Autodesk Fusion 360 part; units mm, degrees
(part 11 of 15)
  spline S48 degree 5 poles (7.9532, 21.0514) (7.9591, 21.034) (7.9709, 20.999) (7.9884, 20.9466) (8.0117, 20.8767) (8.0404, 20.7893) (8.0688, 20.7018) (8.0969, 20.6143) (8.1247, 20.5268) (8.1522, 20.4393) (8.1794, 20.3517) (8.2063, 20.2641) (8.2329, 20.1765) (8.2592, 20.0889) (8.2851, 20.0012) (8.3107, 19.9135) (8.336, 19.8258) (8.361, 19.7381) (8.3856, 19.6503) (8.41, 19.5626) (8.4339, 19.4747) (8.4576, 19.3869) (8.4809, 19.2991) (8.5039, 19.2112) (8.5265, 19.1233) (8.5488, 19.0354) (8.5707, 18.9475) (8.5923, 18.8596) (8.6135, 18.7716) (8.6343, 18.6836) (8.6548, 18.5957) (8.675, 18.5077) (8.6947, 18.4196) (8.7141, 18.3316) (8.7331, 18.2436) (8.7517, 18.1555) (8.7699, 18.0674) (8.7878, 17.9794) (8.8052, 17.8913) (8.8222, 17.8032) (8.8388, 17.7151) (8.855, 17.627) (8.8695, 17.5461) (8.8806, 17.4828) (8.8884, 17.4371) (8.8932, 17.409) (8.895, 17.3986) knots -1 -1 -1 -1 -1 -1 -0.985714 -0.971429 -0.957143 -0.942857 -0.928571 -0.914286 -0.9 -0.885714 -0.871429 -0.857143 -0.842857 -0.828571 -0.814286 -0.8 -0.785714 -0.771429 -0.757143 -0.742857 -0.728571 -0.714286 -0.7 -0.685714 -0.671429 -0.657143 -0.642857 -0.628571 -0.614286 -0.6 -0.585714 -0.571429 -0.557143 -0.542857 -0.528571 -0.514286 -0.5 -0.485714 -0.471429 -0.457143 -0.442857 -0.428571 -0.414286 -0.405839 -0.405839 -0.405839 -0.405839 -0.405839 -0.405839
  arc A48 (10.2055, 17.2577) -> (8.895, 17.3986) centre (2.0032, -52.8695) ccw
  spline S49 degree 5 poles (10.2055, 17.2577) (10.2095, 17.2675) (10.2201, 17.2939) (10.2374, 17.3369) (10.2617, 17.3964) (10.2931, 17.4724) (10.3276, 17.555) (10.3626, 17.6376) (10.398, 17.72) (10.4337, 17.8024) (10.4699, 17.8847) (10.5064, 17.9669) (10.5433, 18.0489) (10.5806, 18.1309) (10.6182, 18.2128) (10.6562, 18.2946) (10.6946, 18.3764) (10.7333, 18.458) (10.7724, 18.5395) (10.8118, 18.6209) (10.8516, 18.7023) (10.8917, 18.7835) (10.9322, 18.8647) (10.973, 18.9458) (11.0141, 19.0267) (11.0555, 19.1076) (11.0973, 19.1884) (11.1394, 19.2691) (11.1818, 19.3497) (11.2246, 19.4302) (11.2676, 19.5106) (11.311, 19.591) (11.3547, 19.6712) (11.3986, 19.7514) (11.4429, 19.8314) (11.4875, 19.9114) (11.5324, 19.9913) (11.5776, 20.071) (11.6231, 20.1507) (11.6689, 20.2303) (11.7149, 20.3098) (11.7613, 20.3892) (11.808, 20.4685) (11.8455, 20.5319) (11.8738, 20.5794) (11.8927, 20.6111) (11.9022, 20.6269) knots 0.405839 0.405839 0.405839 0.405839 0.405839 0.405839 0.414286 0.428571 0.442857 0.457143 0.471429 0.485714 0.5 0.514286 0.528571 0.542857 0.557143 0.571429 0.585714 0.6 0.614286 0.628571 0.642857 0.657143 0.671429 0.685714 0.7 0.714286 0.728571 0.742857 0.757143 0.771429 0.785714 0.8 0.814286 0.828571 0.842857 0.857143 0.871429 0.885714 0.9 0.914286 0.928571 0.942857 0.957143 0.971429 0.985714 1 1 1 1 1 1
  arc A49 (13.2115, 20.4386) -> (11.9022, 20.6269) centre (2.0032, -52.8695) ccw
  spline S50 degree 5 poles (13.2115, 20.4386) (13.2162, 20.4208) (13.2254, 20.3851) (13.2392, 20.3316) (13.2573, 20.2602) (13.2798, 20.1709) (13.3019, 20.0817) (13.3237, 19.9924) (13.3452, 19.9031) (13.3664, 19.8138) (13.3873, 19.7246) (13.4078, 19.6353) (13.4281, 19.546) (13.448, 19.4567) (13.4676, 19.3674) (13.4869, 19.2781) (13.5059, 19.1888) (13.5246, 19.0995) (13.5429, 19.0102) (13.5609, 18.921) (13.5785, 18.8317) (13.5959, 18.7424) (13.6128, 18.6531) (13.6295, 18.5638) (13.6458, 18.4745) (13.6617, 18.3853) (13.6773, 18.296) (13.6926, 18.2068) (13.7075, 18.1175) (13.722, 18.0283) (13.7361, 17.9391) (13.7499, 17.8498) (13.7634, 17.7606) (13.7764, 17.6714) (13.7891, 17.5823) (13.8014, 17.4931) (13.8133, 17.404) (13.8248, 17.3149) (13.8359, 17.2257) (13.8466, 17.1367) (13.8569, 17.0476) (13.8667, 16.9586) (13.8754, 16.8768) (13.882, 16.8129) (13.8865, 16.7668) (13.8893, 16.7385) (13.8903, 16.7279) knots -1 -1 -1 -1 -1 -1 -0.985714 -0.971429 -0.957143 -0.942857 -0.928571 -0.914286 -0.9 -0.885714 -0.871429 -0.857143 -0.842857 -0.828571 -0.814286 -0.8 -0.785714 -0.771429 -0.757143 -0.742857 -0.728571 -0.714286 -0.7 -0.685714 -0.671429 -0.657143 -0.642857 -0.628571 -0.614286 -0.6 -0.585714 -0.571429 -0.557143 -0.542857 -0.528571 -0.514286 -0.5 -0.485714 -0.471429 -0.457143 -0.442857 -0.428571 -0.414286 -0.405839 -0.405839 -0.405839 -0.405839 -0.405839 -0.405839
  arc A50 (15.1874, 16.4939) -> (13.8903, 16.7279) centre (2.0032, -52.8695) ccw
  spline S51 degree 5 poles (15.1874, 16.4939) (15.1921, 16.5034) (15.2045, 16.529) (15.2249, 16.5706) (15.2534, 16.6282) (15.2901, 16.7018) (15.3305, 16.7817) (15.3712, 16.8616) (15.4124, 16.9413) (15.4539, 17.0209) (15.4958, 17.1004) (15.5381, 17.1798) (15.5808, 17.259) (15.6238, 17.3381) (15.6672, 17.4171) (15.711, 17.496) (15.7551, 17.5748) (15.7995, 17.6534) (15.8443, 17.732) (15.8895, 17.8104) (15.9349, 17.8887) (15.9808, 17.9669) (16.0269, 18.0449) (16.0734, 18.1229) (16.1202, 18.2007) (16.1673, 18.2784) (16.2147, 18.356) (16.2624, 18.4335) (16.3105, 18.5109) (16.3589, 18.5882) (16.4076, 18.6653) (16.4565, 18.7423) (16.5058, 18.8193) (16.5554, 18.8961) (16.6053, 18.9728) (16.6555, 19.0493) (16.706, 19.1258) (16.7567, 19.2022) (16.8078, 19.2784) (16.8591, 19.3545) (16.9108, 19.4305) (16.9627, 19.5064) (17.0149, 19.5822) (17.0568, 19.6428) (17.0884, 19.6881) (17.1096, 19.7183) (17.1202, 19.7334) knots 0.405839 0.405839 0.405839 0.405839 0.405839 0.405839 0.414286 0.428571 0.442857 0.457143 0.471429 0.485714 0.5 0.514286 0.528571 0.542857 0.557143 0.571429 0.585714 0.6 0.614286 0.628571 0.642857 0.657143 0.671429 0.685714 0.7 0.714286 0.728571 0.742857 0.757143 0.771429 0.785714 0.8 0.814286 0.828571 0.842857 0.857143 0.871429 0.885714 0.9 0.914286 0.928571 0.942857 0.957143 0.971429 0.985714 1 1 1 1 1 1
  arc A51 (18.4127, 19.4523) -> (17.1202, 19.7334) centre (2.0032, -52.8695) ccw
  spline S52 degree 5 poles (18.4127, 19.4523) (18.4161, 19.4341) (18.4227, 19.3979) (18.4326, 19.3435) (18.4457, 19.271) (18.4617, 19.1804) (18.4774, 19.0897) (18.4927, 18.9992) (18.5078, 18.9086) (18.5226, 18.818) (18.537, 18.7275) (18.5512, 18.637) (18.565, 18.5465) (18.5786, 18.456) (18.5918, 18.3655) (18.6046, 18.2751) (18.6172, 18.1846) (18.6294, 18.0942) (18.6413, 18.0039) (18.6529, 17.9135) (18.6641, 17.8232) (18.6751, 17.7329) (18.6856, 17.6426) (18.6959, 17.5524) (18.7057, 17.4622) (18.7153, 17.372) (18.7245, 17.2819) (18.7333, 17.1918) (18.7418, 17.1017) (18.7499, 17.0116) (18.7577, 16.9216) (18.7651, 16.8317) (18.7721, 16.7417) (18.7788, 16.6518) (18.785, 16.562) (18.7909, 16.4722) (18.7964, 16.3824) (18.8015, 16.2927) (18.8063, 16.203) (18.8106, 16.1134) (18.8145, 16.0238) (18.818, 15.9343) (18.8208, 15.8522) (18.8228, 15.7879) (18.824, 15.7416) (18.8248, 15.7132) (18.825, 15.7026) knots -1 -1 -1 -1 -1 -1 -0.985714 -0.971429 -0.957143 -0.942857 -0.928571 -0.914286 -0.9 -0.885714 -0.871429 -0.857143 -0.842857 -0.828571 -0.814286 -0.8 -0.785714 -0.771429 -0.757143 -0.742857 -0.728571 -0.714286 -0.7 -0.685714 -0.671429 -0.657143 -0.642857 -0.628571 -0.614286 -0.6 -0.585714 -0.571429 -0.557143 -0.542857 -0.528571 -0.514286 -0.5 -0.485714 -0.471429 -0.457143 -0.442857 -0.428571 -0.414286 -0.405839 -0.405839 -0.405839 -0.405839 -0.405839 -0.405839
  arc A52 (20.1022, 15.3766) -> (18.825, 15.7026) centre (2.0032, -52.8695) ccw
  spline S53 degree 5 poles (20.1022, 15.3766) (20.1075, 15.3858) (20.1217, 15.4104) (20.145, 15.4504) (20.1775, 15.5059) (20.2194, 15.5766) (20.2654, 15.6535) (20.3117, 15.7303) (20.3585, 15.8068) (20.4056, 15.8833) (20.4531, 15.9596) (20.5009, 16.0357) (20.5491, 16.1117) (20.5977, 16.1876) (20.6466, 16.2633) (20.6959, 16.3388) (20.7455, 16.4143) (20.7954, 16.4895) (20.8457, 16.5647) (20.8963, 16.6397) (20.9473, 16.7145) (20.9985, 16.7892) (21.0501, 16.8638) (21.102, 16.9383) (21.1543, 17.0126) (21.2068, 17.0867) (21.2597, 17.1607) (21.3128, 17.2346) (21.3663, 17.3084) (21.42, 17.382) (21.4741, 17.4555) (21.5284, 17.5288) (21.5831, 17.602) (21.638, 17.6751) (21.6933, 17.748) (21.7488, 17.8208) (21.8046, 17.8935) (21.8607, 17.966) (21.917, 18.0384) (21.9737, 18.1107) (22.0306, 18.1828) (22.0878, 18.2548) (22.1453, 18.3267) (22.1914, 18.3841) (22.2262, 18.4271) (22.2494, 18.4557) (22.2611, 18.47) knots 0.405839 0.405839 0.405839 0.405839 0.405839 0.405839 0.414286 0.428571 0.442857 0.457143 0.471429 0.485714 0.5 0.514286 0.528571 0.542857 0.557143 0.571429 0.585714 0.6 0.614286 0.628571 0.642857 0.657143 0.671429 0.685714 0.7 0.714286 0.728571 0.742857 0.757143 0.771429 0.785714 0.8 0.814286 0.828571 0.842857 0.857143 0.871429 0.885714 0.9 0.914286 0.928571 0.942857 0.957143 0.971429 0.985714 1 1 1 1 1 1
  arc A53 (23.5303, 18.0974) -> (22.2611, 18.47) centre (2.0032, -52.8695) ccw
  spline S54 degree 5 poles (23.5303, 18.0974) (23.5323, 18.079) (23.5364, 18.0424) (23.5424, 17.9874) (23.5502, 17.9142) (23.5597, 17.8226) (23.5689, 17.7312) (23.5778, 17.6397) (23.5864, 17.5483) (23.5946, 17.4569) (23.6026, 17.3655) (23.6102, 17.2742) (23.6176, 17.183) (23.6246, 17.0918) (23.6313, 17.0006) (23.6377, 16.9095) (23.6438, 16.8184) (23.6496, 16.7273) (23.655, 16.6363) (23.6601, 16.5454) (23.6649, 16.4545) (23.6693, 16.3637) (23.6734, 16.2729) (23.6772, 16.1821) (23.6806, 16.0914) (23.6837, 16.0008) (23.6864, 15.9102) (23.6888, 15.8197) (23.6908, 15.7293) (23.6925, 15.6389) (23.6938, 15.5486) (23.6948, 15.4583) (23.6954, 15.3681) (23.6956, 15.2779) (23.6955, 15.1879) (23.6949, 15.0979) (23.694, 15.0079) (23.6927, 14.9181) (23.691, 14.8283) (23.6889, 14.7386) (23.6864, 14.649) (23.6836, 14.5594) (23.6805, 14.4773) (23.6779, 14.4131) (23.6758, 14.3668) (23.6745, 14.3384) (23.674, 14.3278) knots -1 -1 -1 -1 -1 -1 -0.985714 -0.971429 -0.957143 -0.942857 -0.928571 -0.914286 -0.9 -0.885714 -0.871429 -0.857143 -0.842857 -0.828571 -0.814286 -0.8 -0.785714 -0.771429 -0.757143 -0.742857 -0.728571 -0.714286 -0.7 -0.685714 -0.671429 -0.657143 -0.642857 -0.628571 -0.614286 -0.6 -0.585714 -0.571429 -0.557143 -0.542857 -0.528571 -0.514286 -0.5 -0.485714 -0.471429 -0.457143 -0.442857 -0.428571 -0.414286 -0.405839 -0.405839 -0.405839 -0.405839 -0.405839 -0.405839
  arc A54 (24.9247, 13.9116) -> (23.674, 14.3278) centre (2.0032, -52.8695) ccw
  spline S55 degree 5 poles (24.9247, 13.9116) (24.9306, 13.9203) (24.9466, 13.9439) (24.9727, 13.9821) (25.0091, 14.0351) (25.0559, 14.1027) (25.1072, 14.1761) (25.1589, 14.2494) (25.211, 14.3224) (25.2635, 14.3953) (25.3163, 14.468) (25.3694, 14.5405) (25.4229, 14.6129) (25.4768, 14.6851) (25.531, 14.7571) (25.5855, 14.829) (25.6404, 14.9007) (25.6956, 14.9722) (25.7511, 15.0436) (25.8069, 15.1148) (25.8631, 15.1858) (25.9195, 15.2566) (25.9763, 15.3274) (26.0334, 15.3979) (26.0908, 15.4683) (26.1485, 15.5385) (26.2065, 15.6086) (26.2648, 15.6785) (26.3234, 15.7482) (26.3822, 15.8178) (26.4414, 15.8872) (26.5009, 15.9565) (26.5606, 16.0256) (26.6206, 16.0946) (26.6809, 16.1634) (26.7415, 16.2321) (26.8023, 16.3006) (26.8634, 16.3689) (26.9248, 16.4371) (26.9865, 16.5052) (27.0484, 16.5731) (27.1106, 16.6408) (27.173, 16.7084) (27.2232, 16.7623) (27.2609, 16.8027) (27.2861, 16.8296) (27.2988, 16.8431) knots 0.405839 0.405839 0.405839 0.405839 0.405839 0.405839 0.414286 0.428571 0.442857 0.457143 0.471429 0.485714 0.5 0.514286 0.528571 0.542857 0.557143 0.571429 0.585714 0.6 0.614286 0.628571 0.642857 0.657143 0.671429 0.685714 0.7 0.714286 0.728571 0.742857 0.757143 0.771429 0.785714 0.8 0.814286 0.828571 0.842857 0.857143 0.871429 0.885714 0.9 0.914286 0.928571 0.942857 0.957143 0.971429 0.985714 1 1 1 1 1 1
  arc A55 (28.5381, 16.3808) -> (27.2988, 16.8431) centre (2.0032, -52.8695) ccw
  spline S56 degree 5 poles (28.5381, 16.3808) (28.5389, 16.3624) (28.5403, 16.3256) (28.5424, 16.2703) (28.545, 16.1967) (28.5479, 16.1047) (28.5505, 16.0128) (28.5529, 15.9209) (28.5549, 15.8291) (28.5566, 15.7374) (28.5581, 15.6457) (28.5592, 15.5541) (28.56, 15.4625) (28.5605, 15.3711) (28.5607, 15.2796) (28.5606, 15.1883) (28.5601, 15.097) (28.5594, 15.0058) (28.5583, 14.9146) (28.5569, 14.8236) (28.5552, 14.7326) (28.5531, 14.6416) (28.5507, 14.5508) (28.548, 14.46) (28.545, 14.3693) (28.5416, 14.2787) (28.5379, 14.1881) (28.5338, 14.0977) (28.5294, 14.0073) (28.5246, 13.917) (28.5195, 13.8268) (28.514, 13.7367) (28.5081, 13.6467) (28.5019, 13.5568) (28.4953, 13.467) (28.4884, 13.3772) (28.4811, 13.2876) (28.4734, 13.1981) (28.4653, 13.1086) (28.4568, 13.0193) (28.4479, 12.9301) (28.4386, 12.841) (28.4298, 12.7593) (28.4225, 12.6954) (28.4172, 12.6494) (28.4139, 12.6211) (28.4126, 12.6106) knots -1 -1 -1 -1 -1 -1 -0.985714 -0.971429 -0.957143 -0.942857 -0.928571 -0.914286 -0.9 -0.885714 -0.871429 -0.857143 -0.842857 -0.828571 -0.814286 -0.8 -0.785714 -0.771429 -0.757143 -0.742857 -0.728571 -0.714286 -0.7 -0.685714 -0.671429 -0.657143 -0.642857 -0.628571 -0.614286 -0.6 -0.585714 -0.571429 -0.557143 -0.542857 -0.528571 -0.514286 -0.5 -0.485714 -0.471429 -0.457143 -0.442857 -0.428571 -0.414286 -0.405839 -0.405839 -0.405839 -0.405839 -0.405839 -0.405839
  arc A56 (29.6304, 12.1062) -> (28.4126, 12.6106) centre (2.0032, -52.8695) ccw
  spline S57 degree 5 poles (29.6304, 12.1062) (29.6369, 12.1145) (29.6545, 12.1369) (29.6833, 12.1732) (29.7234, 12.2234) (29.7749, 12.2875) (29.8313, 12.3571) (29.8881, 12.4264) (29.9453, 12.4956) (30.0028, 12.5646) (30.0607, 12.6333) (30.1189, 12.7019) (30.1774, 12.7702) (30.2363, 12.8384) (30.2955, 12.9064) (30.355, 12.9742) (30.4148, 13.0418) (30.475, 13.1092) (30.5354, 13.1764) (30.5962, 13.2434) (30.6573, 13.3102) (30.7187, 13.3769) (30.7804, 13.4434) (30.8423, 13.5097) (30.9046, 13.5758) (30.9672, 13.6417) (31.03, 13.7075) (31.0931, 13.773) (31.1565, 13.8384) (31.2202, 13.9036) (31.2842, 13.9687) (31.3484, 14.0335) (31.4129, 14.0982) (31.4777, 14.1627) (31.5428, 14.227) (31.6081, 14.2912) (31.6737, 14.3552) (31.7395, 14.419) (31.8056, 14.4827) (31.8719, 14.5461) (31.9385, 14.6094) (32.0054, 14.6726) (32.0725, 14.7355) (32.1264, 14.7858) (32.1669, 14.8234) (32.194, 14.8484) (32.2075, 14.8609) knots 0.405839 0.405839 0.405839 0.405839 0.405839 0.405839 0.414286 0.428571 0.442857 0.457143 0.471429 0.485714 0.5 0.514286 0.528571 0.542857 0.557143 0.571429 0.585714 0.6 0.614286 0.628571 0.642857 0.657143 0.671429 0.685714 0.7 0.714286 0.728571 0.742857 0.757143 0.771429 0.785714 0.8 0.814286 0.828571 0.842857 0.857143 0.871429 0.885714 0.9 0.914286 0.928571 0.942857 0.957143 0.971429 0.985714 1 1 1 1 1 1
  arc A57 (33.4108, 14.3114) -> (32.2075, 14.8609) centre (2.0032, -52.8695) ccw
  spline S58 degree 5 poles (33.4108, 14.3114) (33.4102, 14.293) (33.409, 14.2561) (33.4071, 14.2009) (33.4045, 14.1272) (33.4008, 14.0353) (33.3969, 13.9434) (33.3927, 13.8516) (33.3882, 13.7599) (33.3833, 13.6683) (33.3782, 13.5767) (33.3728, 13.4853) (33.3671, 13.3939) (33.3611, 13.3026) (33.3547, 13.2114) (33.3481, 13.1203) (33.3412, 13.0293) (33.3339, 12.9383) (33.3263, 12.8475) (33.3184, 12.7568) (33.3102, 12.6661) (33.3017, 12.5756) (33.2928, 12.4851) (33.2836, 12.3948) (33.2741, 12.3045) (33.2643, 12.2144) (33.2541, 12.1243) (33.2436, 12.0344) (33.2327, 11.9446) (33.2215, 11.8549) (33.21, 11.7653) (33.1981, 11.6758) (33.1858, 11.5864) (33.1732, 11.4972) (33.1602, 11.408) (33.1469, 11.319) (33.1332, 11.2301) (33.1191, 11.1414) (33.1047, 11.0528) (33.0898, 10.9643) (33.0746, 10.8759) (33.059, 10.7877) (33.0443, 10.7068) (33.0326, 10.6436) (33.024, 10.5981) (33.0186, 10.5702) (33.0166, 10.5598) knots -1 -1 -1 -1 -1 -1 -0.985714 -0.971429 -0.957143 -0.942857 -0.928571 -0.914286 -0.9 -0.885714 -0.871429 -0.857143 -0.842857 -0.828571 -0.814286 -0.8 -0.785714 -0.771429 -0.757143 -0.742857 -0.728571 -0.714286 -0.7 -0.685714 -0.671429 -0.657143 -0.642857 -0.628571 -0.614286 -0.6 -0.585714 -0.571429 -0.557143 -0.542857 -0.528571 -0.514286 -0.5 -0.485714 -0.471429 -0.457143 -0.442857 -0.428571 -0.414286 -0.405839 -0.405839 -0.405839 -0.405839 -0.405839 -0.405839
  arc A58 (34.1953, 9.9698) -> (33.0166, 10.5598) centre (2.0032, -52.8695) ccw
  spline S59 degree 5 poles (34.1953, 9.9698) (34.2024, 9.9776) (34.2216, 9.9986) (34.2529, 10.0328) (34.2964, 10.0801) (34.3524, 10.1403) (34.4136, 10.2057) (34.4752, 10.2708) (34.5372, 10.3357) (34.5995, 10.4004) (34.6621, 10.4648) (34.725, 10.5291) (34.7883, 10.5931) (34.8519, 10.6569) (34.9158, 10.7204) (34.98, 10.7838) (35.0445, 10.847) (35.1093, 10.9099) (35.1744, 10.9726) (35.2398, 11.0352) (35.3055, 11.0975) (35.3715, 11.1596) (35.4377, 11.2215) (35.5043, 11.2832) (35.5711, 11.3447) (35.6382, 11.406) (35.7056, 11.4671) (35.7732, 11.528) (35.8411, 11.5887) (35.9093, 11.6492) (35.9778, 11.7095) (36.0465, 11.7696) (36.1154, 11.8295) (36.1846, 11.8892) (36.2541, 11.9488) (36.3238, 12.0081) (36.3938, 12.0673) (36.464, 12.1262) (36.5345, 12.185) (36.6052, 12.2436) (36.6762, 12.3019) (36.7474, 12.3601) (36.8188, 12.4182) (36.8761, 12.4644) (36.9192, 12.499) (36.948, 12.5221) (36.9624, 12.5336) knots 0.405839 0.405839 0.405839 0.405839 0.405839 0.405839 0.414286 0.428571 0.442857 0.457143 0.471429 0.485714 0.5 0.514286 0.528571 0.542857 0.557143 0.571429 0.585714 0.6 0.614286 0.628571 0.642857 0.657143 0.671429 0.685714 0.7 0.714286 0.728571 0.742857 0.757143 0.771429 0.785714 0.8 0.814286 0.828571 0.842857 0.857143 0.871429 0.885714 0.9 0.914286 0.928571 0.942857 0.957143 0.971429 0.985714 1 1 1 1 1 1
  arc A59 (38.1234, 11.8996) -> (36.9624, 12.5336) centre (2.0032, -52.8695) ccw
  spline S60 degree 5 poles (38.1234, 11.8996) (38.1215, 11.8813) (38.1177, 11.8446) (38.1119, 11.7896) (38.1039, 11.7164) (38.0938, 11.6249) (38.0833, 11.5336) (38.0725, 11.4423) (38.0615, 11.3512) (38.0501, 11.2601) (38.0385, 11.1692) (38.0266, 11.0783) (38.0144, 10.9876) (38.0018, 10.897) (37.989, 10.8065) (37.9759, 10.716) (37.9625, 10.6258) (37.9487, 10.5356) (37.9347, 10.4455) (37.9204, 10.3556) (37.9057, 10.2657) (37.8907, 10.176) (37.8754, 10.0864) (37.8598, 9.997) (37.8439, 9.9076) (37.8276, 9.8184) (37.8111, 9.7293) (37.7942, 9.6404) (37.7769, 9.5515) (37.7593, 9.4629) (37.7414, 9.3743) (37.7232, 9.2859) (37.7046, 9.1976) (37.6856, 9.1095) (37.6663, 9.0215) (37.6467, 8.9337) (37.6267, 8.846) (37.6063, 8.7585) (37.5856, 8.6711) (37.5645, 8.5839) (37.543, 8.4969) (37.5211, 8.41) (37.5007, 8.3304) (37.4845, 8.2682) (37.4726, 8.2234) (37.4653, 8.1959) (37.4626, 8.1857) knots -1 -1 -1 -1 -1 -1 -0.985714 -0.971429 -0.957143 -0.942857 -0.928571 -0.914286 -0.9 -0.885714 -0.871429 -0.857143 -0.842857 -0.828571 -0.814286 -0.8 -0.785714 -0.771429 -0.757143 -0.742857 -0.728571 -0.714286 -0.7 -0.685714 -0.671429 -0.657143 -0.642857 -0.628571 -0.614286 -0.6 -0.585714 -0.571429 -0.557143 -0.542857 -0.528571 -0.514286 -0.5 -0.485714 -0.471429 -0.457143 -0.442857 -0.428571 -0.414286 -0.405839 -0.405839 -0.405839 -0.405839 -0.405839 -0.405839
  arc A60 (38.5962, 7.5131) -> (37.4626, 8.1857) centre (2.0032, -52.8695) ccw
  spline S61 degree 5 poles (38.5962, 7.5131) (38.6038, 7.5204) (38.6245, 7.54) (38.6581, 7.5719) (38.7049, 7.6159) (38.765, 7.672) (38.8308, 7.7328) (38.8969, 7.7934) (38.9633, 7.8537) (39.03, 7.9138) (39.0971, 7.9736) (39.1645, 8.0332) (39.2321, 8.0925) (39.3001, 8.1516) (39.3684, 8.2105) (39.4369, 8.2691) (39.5058, 8.3275) (39.5749, 8.3856) (39.6443, 8.4436) (39.714, 8.5013) (39.784, 8.5587) (39.8542, 8.616) (39.9247, 8.673) (39.9955, 8.7298) (40.0666, 8.7864) (40.1379, 8.8427) (40.2094, 8.8989) (40.2812, 8.9548) (40.3533, 9.0105) (40.4256, 9.066) (40.4982, 9.1212) (40.571, 9.1763) (40.6441, 9.2311) (40.7174, 9.2858) (40.7909, 9.3402) (40.8647, 9.3944) (40.9387, 9.4484) (41.013, 9.5022) (41.0875, 9.5558) (41.1622, 9.6092) (41.2371, 9.6624) (41.3123, 9.7153) (41.3876, 9.7681) (41.4481, 9.8101) (41.4936, 9.8416) (41.524, 9.8625) (41.5391, 9.873) knots 0.405839 0.405839 0.405839 0.405839 0.405839 0.405839 0.414286 0.428571 0.442857 0.457143 0.471429 0.485714 0.5 0.514286 0.528571 0.542857 0.557143 0.571429 0.585714 0.6 0.614286 0.628571 0.642857 0.657143 0.671429 0.685714 0.7 0.714286 0.728571 0.742857 0.757143 0.771429 0.785714 0.8 0.814286 0.828571 0.842857 0.857143 0.871429 0.885714 0.9 0.914286 0.928571 0.942857 0.957143 0.971429 0.985714 1 1 1 1 1 1
  arc A61 (42.6519, 9.1578) -> (41.5391, 9.873) centre (2.0032, -52.8695) ccw
  spline S62 degree 5 poles (42.6519, 9.1578) (42.6487, 9.1397) (42.6423, 9.1034) (42.6326, 9.0489) (42.6195, 8.9764) (42.6028, 8.886) (42.5858, 8.7956) (42.5686, 8.7053) (42.5511, 8.6152) (42.5332, 8.5252) (42.5152, 8.4353) (42.4968, 8.3455) (42.4781, 8.2559) (42.4592, 8.1664) (42.4399, 8.077) (42.4204, 7.9878) (42.4005, 7.8987) (42.3804, 7.8097) (42.36, 7.7209) (42.3393, 7.6322) (42.3182, 7.5436) (42.2969, 7.4552) (42.2753, 7.3669) (42.2533, 7.2788) (42.231, 7.1908) (42.2085, 7.103) (42.1856, 7.0153) (42.1624, 6.9278) (42.1388, 6.8404) (42.115, 6.7532) (42.0908, 6.6662) (42.0663, 6.5793) (42.0414, 6.4926) (42.0163, 6.406) (41.9907, 6.3197) (41.9649, 6.2335) (41.9387, 6.1474) (41.9121, 6.0616) (41.8852, 5.9759) (41.8579, 5.8904) (41.8303, 5.8051) (41.8023, 5.72) (41.7762, 5.6421) (41.7556, 5.5812) (41.7406, 5.5374) (41.7313, 5.5105) (41.7279, 5.5005) knots -1 -1 -1 -1 -1 -1 -0.985714 -0.971429 -0.957143 -0.942857 -0.928571 -0.914286 -0.9 -0.885714 -0.871429 -0.857143 -0.842857 -0.828571 -0.814286 -0.8 -0.785714 -0.771429 -0.757143 -0.742857 -0.728571 -0.714286 -0.7 -0.685714 -0.671429 -0.657143 -0.642857 -0.628571 -0.614286 -0.6 -0.585714 -0.571429 -0.557143 -0.542857 -0.528571 -0.514286 -0.5 -0.485714 -0.471429 -0.457143 -0.442857 -0.428571 -0.414286 -0.405839 -0.405839 -0.405839 -0.405839 -0.405839 -0.405839
  arc A62 (42.8106, 4.7487) -> (41.7279, 5.5005) centre (2.0032, -52.8695) ccw
  spline S63 degree 5 poles (42.8106, 4.7487) (42.8188, 4.7555) (42.8407, 4.7736) (42.8766, 4.8029) (42.9264, 4.8435) (42.9903, 4.8952) (43.0603, 4.9512) (43.1305, 5.0069) (43.2011, 5.0623) (43.2719, 5.1174) (43.3431, 5.1723) (43.4145, 5.2269) (43.4863, 5.2813) (43.5583, 5.3354) (43.6306, 5.3892) (43.7031, 5.4428) (43.776, 5.4962) (43.8491, 5.5492) (43.9224, 5.6021) (43.9961, 5.6546) (44.07, 5.707) (44.1441, 5.7591) (44.2185, 5.8109) (44.2932, 5.8625) (44.3681, 5.9139) (44.4432, 5.965) (44.5186, 6.0159) (44.5942, 6.0665) (44.6701, 6.1169) (44.7462, 6.1671) (44.8225, 6.2171) (44.8991, 6.2668) (44.9758, 6.3163) (45.0529, 6.3656) (45.1301, 6.4146) (45.2075, 6.4634) (45.2852, 6.512) (45.3631, 6.5604) (45.4412, 6.6085) (45.5196, 6.6564) (45.5981, 6.7041) (45.6769, 6.7516) (45.7558, 6.7988) (45.8191, 6.8365) (45.8667, 6.8646) (45.8985, 6.8833) (45.9144, 6.8927) knots 0.405839 0.405839 0.405839 0.405839 0.405839 0.405839 0.414286 0.428571 0.442857 0.457143 0.471429 0.485714 0.5 0.514286 0.528571 0.542857 0.557143 0.571429 0.585714 0.6 0.614286 0.628571 0.642857 0.657143 0.671429 0.685714 0.7 0.714286 0.728571 0.742857 0.757143 0.771429 0.785714 0.8 0.814286 0.828571 0.842857 0.857143 0.871429 0.885714 0.9 0.914286 0.928571 0.942857 0.957143 0.971429 0.985714 1 1 1 1 1 1
  arc A63 (46.9733, 6.0999) -> (45.9144, 6.8927) centre (2.0032, -52.8695) ccw
  spline S64 degree 5 poles (46.9733, 6.0999) (46.9689, 6.0821) (46.9599, 6.0463) (46.9463, 5.9927) (46.928, 5.9213) (46.9049, 5.8323) (46.8816, 5.7433) (46.8579, 5.6545) (46.834, 5.5659) (46.8098, 5.4774) (46.7854, 5.389) (46.7606, 5.3008) (46.7356, 5.2127) (46.7103, 5.1248) (46.6848, 5.037) (46.6589, 4.9494) (46.6328, 4.8619) (46.6063, 4.7746) (46.5796, 4.6875) (46.5526, 4.6005) (46.5253, 4.5136) (46.4977, 4.427) (46.4699, 4.3405) (46.4417, 4.2541) (46.4132, 4.168) (46.3844, 4.082) (46.3553, 3.9962) (46.3259, 3.9105) (46.2962, 3.8251) (46.2662, 3.7398) (46.2359, 3.6547) (46.2052, 3.5698) (46.1743, 3.485) (46.143, 3.4005) (46.1114, 3.3162) (46.0794, 3.232) (46.0471, 3.1481) (46.0145, 3.0644) (45.9816, 2.9808) (45.9483, 2.8975) (45.9146, 2.8144) (45.8806, 2.7315) (45.849, 2.6556) (45.8241, 2.5964) (45.806, 2.5537) (45.7949, 2.5276) (45.7907, 2.5179) knots -1 -1 -1 -1 -1 -1 -0.985714 -0.971429 -0.957143 -0.942857 -0.928571 -0.914286 -0.9 -0.885714 -0.871429 -0.857143 -0.842857 -0.828571 -0.814286 -0.8 -0.785714 -0.771429 -0.757143 -0.742857 -0.728571 -0.714286 -0.7 -0.685714 -0.671429 -0.657143 -0.642857 -0.628571 -0.614286 -0.6 -0.585714 -0.571429 -0.557143 -0.542857 -0.528571 -0.514286 -0.5 -0.485714 -0.471429 -0.457143 -0.442857 -0.428571 -0.414286 -0.405839 -0.405839 -0.405839 -0.405839 -0.405839 -0.405839
  arc A64 (46.8171, 1.6908) -> (45.7907, 2.5179) centre (2.0032, -52.8695) ccw
  spline S65 degree 5 poles (46.8171, 1.6908) (46.8257, 1.6969) (46.8489, 1.7134) (46.8867, 1.7401) (46.9393, 1.7771) (47.0068, 1.824) (47.0805, 1.8749) (47.1546, 1.9254) (47.2289, 1.9757) (47.3035, 2.0256) (47.3784, 2.0753) (47.4536, 2.1247) (47.529, 2.1738) (47.6047, 2.2226) (47.6806, 2.2711) (47.7568, 2.3194) (47.8333, 2.3674) (47.91, 2.4151) (47.987, 2.4626) (48.0641, 2.5098) (48.1416, 2.5567) (48.2193, 2.6034) (48.2972, 2.6498) (48.3753, 2.6959) (48.4537, 2.7418) (48.5323, 2.7874) (48.6111, 2.8328) (48.6901, 2.878) (48.7694, 2.9228) (48.8489, 2.9675) (48.9286, 3.0118) (49.0085, 3.056) (49.0886, 3.0999) (49.1689, 3.1435) (49.2495, 3.1869) (49.3302, 3.2301) (49.4112, 3.273) (49.4923, 3.3157) (49.5737, 3.3581) (49.6552, 3.4003) (49.737, 3.4423) (49.8189, 3.484) (49.901, 3.5255) (49.9669, 3.5586) (50.0164, 3.5832) (50.0494, 3.5996) (50.0659, 3.6078) knots 0.405839 0.405839 0.405839 0.405839 0.405839 0.405839 0.414286 0.428571 0.442857 0.457143 0.471429 0.485714 0.5 0.514286 0.528571 0.542857 0.557143 0.571429 0.585714 0.6 0.614286 0.628571 0.642857 0.657143 0.671429 0.685714 0.7 0.714286 0.728571 0.742857 0.757143 0.771429 0.785714 0.8 0.814286 0.828571 0.842857 0.857143 0.871429 0.885714 0.9 0.914286 0.928571 0.942857 0.957143 0.971429 0.985714 1 1 1 1 1 1
  arc A65 (51.0656, 2.7416) -> (50.0659, 3.6078) centre (2.0032, -52.8695) ccw
  spline S66 degree 5 poles (51.0656, 2.7416) (51.0598, 2.724) (51.0483, 2.689) (51.031, 2.6365) (51.0077, 2.5666) (50.9783, 2.4794) (50.9486, 2.3924) (50.9187, 2.3055) (50.8885, 2.2188) (50.8581, 2.1322) (50.8274, 2.0458) (50.7964, 1.9596) (50.7652, 1.8735) (50.7337, 1.7877) (50.7019, 1.7019) (50.6699, 1.6164) (50.6376, 1.531) (50.605, 1.4458) (50.5721, 1.3608) (50.539, 1.2759) (50.5056, 1.1913) (50.4719, 1.1068) (50.4379, 1.0225) (50.4036, 0.9384) (50.3691, 0.8545) (50.3342, 0.7708) (50.2991, 0.6872) (50.2636, 0.6039) (50.2279, 0.5208) (50.1919, 0.4379) (50.1556, 0.3551) (50.1189, 0.2726) (50.082, 0.1903) (50.0448, 0.1083) (50.0072, 0.0264) (49.9693, -0.0553) (49.9312, -0.1367) (49.8927, -0.2179) (49.8538, -0.2988) (49.8147, -0.3796) (49.7752, -0.4601) (49.7353, -0.5403) (49.6985, -0.6138) (49.6694, -0.6711) (49.6483, -0.7123) (49.6353, -0.7376) (49.6305, -0.747) knots -1 -1 -1 -1 -1 -1 -0.985714 -0.971429 -0.957143 -0.942857 -0.928571 -0.914286 -0.9 -0.885714 -0.871429 -0.857143 -0.842857 -0.828571 -0.814286 -0.8 -0.785714 -0.771429 -0.757143 -0.742857 -0.728571 -0.714286 -0.7 -0.685714 -0.671429 -0.657143 -0.642857 -0.628571 -0.614286 -0.6 -0.585714 -0.571429 -0.557143 -0.542857 -0.528571 -0.514286 -0.5 -0.485714 -0.471429 -0.457143 -0.442857 -0.428571 -0.414286 -0.405839 -0.405839 -0.405839 -0.405839 -0.405839 -0.405839
  arc A66 (50.5952, -1.6452) -> (49.6305, -0.747) centre (2.0032, -52.8695) ccw
  spline S67 degree 5 poles (50.5952, -1.6452) (50.6042, -1.6397) (50.6285, -1.625) (50.6682, -1.601) (50.7232, -1.5679) (50.7939, -1.5259) (50.8711, -1.4804) (50.9486, -1.4353) (51.0263, -1.3904) (51.1043, -1.3459) (51.1825, -1.3017) (51.261, -1.2578) (51.3397, -1.2142) (51.4187, -1.1709) (51.4979, -1.1279) (51.5774, -1.0852) (51.6571, -1.0428) (51.737, -1.0007) (51.8171, -0.9588) (51.8975, -0.9173) (51.9781, -0.876) (52.0589, -0.835) (52.1399, -0.7942) (52.2211, -0.7538) (52.3026, -0.7136) (52.3842, -0.6737) (52.4661, -0.6341) (52.5482, -0.5947) (52.6304, -0.5556) (52.7129, -0.5167) (52.7955, -0.4782) (52.8784, -0.4398) (52.9615, -0.4018) (53.0447, -0.364) (53.1281, -0.3264) (53.2117, -0.2891) (53.2955, -0.2521) (53.3795, -0.2153) (53.4637, -0.1788) (53.548, -0.1425) (53.6326, -0.1065) (53.7173, -0.0707) (53.8022, -0.0351) (53.8702, -0.0069) (53.9213, 0.0142) (53.9554, 0.0282) (53.9725, 0.0351) knots 0.405839 0.405839 0.405839 0.405839 0.405839 0.405839 0.414286 0.428571 0.442857 0.457143 0.471429 0.485714 0.5 0.514286 0.528571 0.542857 0.557143 0.571429 0.585714 0.6 0.614286 0.628571 0.642857 0.657143 0.671429 0.685714 0.7 0.714286 0.728571 0.742857 0.757143 0.771429 0.785714 0.8 0.814286 0.828571 0.842857 0.857143 0.871429 0.885714 0.9 0.914286 0.928571 0.942857 0.957143 0.971429 0.985714 1 1 1 1 1 1
  arc A67 (54.9078, -0.9002) -> (53.9725, 0.0351) centre (2.0032, -52.8695) ccw
  spline S68 degree 5 poles (54.9078, -0.9002) (54.9009, -0.9173) (54.8869, -0.9514) (54.8658, -1.0025) (54.8376, -1.0705) (54.802, -1.1554) (54.7662, -1.2401) (54.7302, -1.3246) (54.6939, -1.409) (54.6574, -1.4932) (54.6206, -1.5772) (54.5836, -1.661) (54.5463, -1.7446) (54.5087, -1.828) (54.4709, -1.9112) (54.4329, -1.9943) (54.3945, -2.0771) (54.356, -2.1598) (54.3171, -2.2423) (54.278, -2.3245) (54.2386, -2.4066) (54.199, -2.4885) (54.1591, -2.5701) (54.1189, -2.6515) (54.0784, -2.7328) (54.0377, -2.8138) (53.9967, -2.8946) (53.9554, -2.9752) (53.9139, -3.0556) (53.872, -3.1357) (53.8299, -3.2156) (53.7875, -3.2953) (53.7448, -3.3748) (53.7018, -3.454) (53.6585, -3.533) (53.6149, -3.6117) (53.571, -3.6902) (53.5268, -3.7684) (53.4822, -3.8464) (53.4374, -3.9241) (53.3923, -4.0016) (53.3468, -4.0788) (53.3048, -4.1495) (53.2717, -4.2045) (53.2477, -4.2442) (53.233, -4.2685) (53.2275, -4.2775) knots -1 -1 -1 -1 -1 -1 -0.985714 -0.971429 -0.957143 -0.942857 -0.928571 -0.914286 -0.9 -0.885714 -0.871429 -0.857143 -0.842857 -0.828571 -0.814286 -0.8 -0.785714 -0.771429 -0.757143 -0.742857 -0.728571 -0.714286 -0.7 -0.685714 -0.671429 -0.657143 -0.642857 -0.628571 -0.614286 -0.6 -0.585714 -0.571429 -0.557143 -0.542857 -0.528571 -0.514286 -0.5 -0.485714 -0.471429 -0.457143 -0.442857 -0.428571 -0.414286 -0.405839 -0.405839 -0.405839 -0.405839 -0.405839 -0.405839
  arc A68 (54.1257, -5.2422) -> (53.2275, -4.2775) centre (2.0032, -52.8695) ccw
  spline S69 degree 5 poles (54.1257, -5.2422) (54.1351, -5.2374) (54.1604, -5.2244) (54.2016, -5.2033) (54.2589, -5.1742) (54.3324, -5.1374) (54.4126, -5.0975) (54.4931, -5.058) (54.5739, -5.0189) (54.6548, -4.98) (54.736, -4.9415) (54.8174, -4.9033) (54.8991, -4.8655) (54.9809, -4.8279) (55.063, -4.7907) (55.1453, -4.7538) (55.2278, -4.7171) (55.3106, -4.6808) (55.3935, -4.6448) (55.4766, -4.6091) (55.5599, -4.5736) (55.6435, -4.5385) (55.7272, -4.5036) (55.8111, -4.4691) (55.8952, -4.4348) (55.9795, -4.4008) (56.064, -4.3671) (56.1486, -4.3337) (56.2335, -4.3006) (56.3185, -4.2677) (56.4037, -4.2351) (56.4891, -4.2028) (56.5746, -4.1708) (56.6603, -4.139) (56.7462, -4.1075) (56.8323, -4.0763) (56.9185, -4.0453) (57.0049, -4.0146) (57.0915, -3.9842) (57.1782, -3.954) (57.2651, -3.9241) (57.3521, -3.8944) (57.4393, -3.865) (57.5092, -3.8417) (57.5617, -3.8244) (57.5967, -3.8128) (57.6143, -3.8071) knots 0.405839 0.405839 0.405839 0.405839 0.405839 0.405839 0.414286 0.428571 0.442857 0.457143 0.471429 0.485714 0.5 0.514286 0.528571 0.542857 0.557143 0.571429 0.585714 0.6 0.614286 0.628571 0.642857 0.657143 0.671429 0.685714 0.7 0.714286 0.728571 0.742857 0.757143 0.771429 0.785714 0.8 0.814286 0.828571 0.842857 0.857143 0.871429 0.885714 0.9 0.914286 0.928571 0.942857 0.957143 0.971429 0.985714 1 1 1 1 1 1
  arc A69 (58.4805, -4.8068) -> (57.6143, -3.8071) centre (2.0032, -52.8695) ccw
  spline S70 degree 5 poles (58.4805, -4.8068) (58.4723, -4.8233) (58.4559, -4.8563) (58.4313, -4.9058) (58.3982, -4.9717) (58.3567, -5.0538) (58.315, -5.1357) (58.273, -5.2175) (58.2308, -5.299) (58.1884, -5.3804) (58.1457, -5.4615) (58.1028, -5.5425) (58.0596, -5.6232) (58.0162, -5.7037) (57.9726, -5.7841) (57.9287, -5.8642) (57.8845, -5.9441) (57.8402, -6.0238) (57.7955, -6.1033) (57.7507, -6.1826) (57.7055, -6.2616) (57.6601, -6.3404) (57.6145, -6.419) (57.5686, -6.4974) (57.5225, -6.5755) (57.4761, -6.6534) (57.4294, -6.7311) (57.3825, -6.8085) (57.3353, -6.8857) (57.2878, -6.9627) (57.2401, -7.0394) (57.1921, -7.1159) (57.1438, -7.1921) (57.0953, -7.268) (57.0465, -7.3437) (56.9974, -7.4191) (56.948, -7.4943) (56.8983, -7.5692) (56.8484, -7.6438) (56.7981, -7.7181) (56.7476, -7.7922) (56.6967, -7.8659) (56.6497, -7.9334) (56.6128, -7.986) (56.5861, -8.0238) (56.5696, -8.047) (56.5635, -8.0556) knots -1 -1 -1 -1 -1 -1 -0.985714 -0.971429 -0.957143 -0.942857 -0.928571 -0.914286 -0.9 -0.885714 -0.871429 -0.857143 -0.842857 -0.828571 -0.814286 -0.8 -0.785714 -0.771429 -0.757143 -0.742857 -0.728571 -0.714286 -0.7 -0.685714 -0.671429 -0.657143 -0.642857 -0.628571 -0.614286 -0.6 -0.585714 -0.571429 -0.557143 -0.542857 -0.528571 -0.514286 -0.5 -0.485714 -0.471429 -0.457143 -0.442857 -0.428571 -0.414286 -0.405839 -0.405839 -0.405839 -0.405839 -0.405839 -0.405839
  arc A70 (57.3905, -9.082) -> (56.5635, -8.0556) centre (2.0032, -52.8695) ccw
  spline S71 degree 5 poles (57.3905, -9.082) (57.4003, -9.0778) (57.4264, -9.0667) (57.4691, -9.0486) (57.5283, -9.0236) (57.6042, -8.9921) (57.6871, -8.9581) (57.7702, -8.9244) (57.8535, -8.8911) (57.9371, -8.8582) (58.0208, -8.8256) (58.1047, -8.7933) (58.1889, -8.7613) (58.2732, -8.7297) (58.3577, -8.6984) (58.4425, -8.6675) (58.5274, -8.6368) (58.6125, -8.6065) (58.6978, -8.5765) (58.7832, -8.5468) (58.8689, -8.5174) (58.9547, -8.4883) (59.0407, -8.4595) (59.1268, -8.431) (59.2132, -8.4028) (59.2997, -8.3749) (59.3863, -8.3474) (59.4732, -8.3201) (59.5602, -8.2931) (59.6473, -8.2664) (59.7346, -8.2399) (59.8221, -8.2138) (59.9097, -8.1879) (59.9975, -8.1624) (60.0854, -8.1371) (60.1735, -8.1121) (60.2617, -8.0873) (60.3501, -8.0629) (60.4386, -8.0387) (60.5272, -8.0148) (60.616, -7.9911) (60.705, -7.9678) (60.794, -7.9447) (60.8654, -7.9264) (60.919, -7.9128) (60.9548, -7.9038) (60.9726, -7.8993) knots 0.405839 0.405839 0.405839 0.405839 0.405839 0.405839 0.414286 0.428571 0.442857 0.457143 0.471429 0.485714 0.5 0.514286 0.528571 0.542857 0.557143 0.571429 0.585714 0.6 0.614286 0.628571 0.642857 0.657143 0.671429 0.685714 0.7 0.714286 0.728571 0.742857 0.757143 0.771429 0.785714 0.8 0.814286 0.828571 0.842857 0.857143 0.871429 0.885714 0.9 0.914286 0.928571 0.942857 0.957143 0.971429 0.985714 1 1 1 1 1 1
  arc A71 (61.7653, -8.9583) -> (60.9726, -7.8993) centre (2.0032, -52.8695) ccw
  spline S72 degree 5 poles (61.7653, -8.9583) (61.756, -8.9742) (61.7373, -9.006) (61.7092, -9.0535) (61.6715, -9.1169) (61.6243, -9.1958) (61.5768, -9.2746) (61.5291, -9.3531) (61.4812, -9.4315) (61.4331, -9.5096) (61.3847, -9.5875) (61.3361, -9.6651) (61.2873, -9.7426) (61.2383, -9.8198) (61.189, -9.8969) (61.1395, -9.9736) (61.0898, -10.0502) (61.0398, -10.1265) (60.9896, -10.2026) (60.9392, -10.2785) (60.8886, -10.3541) (60.8377, -10.4295) (60.7866, -10.5046) (60.7352, -10.5795) (60.6836, -10.6542) (60.6317, -10.7286) (60.5797, -10.8027) (60.5273, -10.8766) (60.4747, -10.9502) (60.4219, -11.0236) (60.3688, -11.0967) (60.3155, -11.1696) (60.2619, -11.2421) (60.2081, -11.3144) (60.154, -11.3864) (60.0996, -11.4582) (60.045, -11.5296) (59.9901, -11.6008) (59.935, -11.6716) (59.8795, -11.7422) (59.8238, -11.8124) (59.7679, -11.8824) (59.7162, -11.9463) (59.6756, -11.9961) (59.6462, -12.032) (59.6282, -12.0539) (59.6214, -12.0621) knots -1 -1 -1 -1 -1 -1 -0.985714 -0.971429 -0.957143 -0.942857 -0.928571 -0.914286 -0.9 -0.885714 -0.871429 -0.857143 -0.842857 -0.828571 -0.814286 -0.8 -0.785714 -0.771429 -0.757143 -0.742857 -0.728571 -0.714286 -0.7 -0.685714 -0.671429 -0.657143 -0.642857 -0.628571 -0.614286 -0.6 -0.585714 -0.571429 -0.557143 -0.542857 -0.528571 -0.514286 -0.5 -0.485714 -0.471429 -0.457143 -0.442857 -0.428571 -0.414286 -0.405839 -0.405839 -0.405839 -0.405839 -0.405839 -0.405839
  arc A72 (60.3732, -13.1448) -> (59.6214, -12.0621) centre (2.0032, -52.8695) ccw
  spline S73 degree 5 poles (60.3732, -13.1448) (60.3832, -13.1414) (60.4101, -13.1321) (60.4539, -13.1171) (60.5148, -13.0965) (60.5927, -13.0704) (60.6778, -13.0424) (60.7631, -13.0148) (60.8486, -12.9875) (60.9343, -12.9606) (61.0201, -12.934) (61.1062, -12.9078) (61.1924, -12.882) (61.2787, -12.8564) (61.3653, -12.8313) (61.452, -12.8064) (61.5389, -12.7819) (61.6259, -12.7577) (61.7131, -12.7339) (61.8005, -12.7103) (61.888, -12.6871) (61.9757, -12.6642) (62.0635, -12.6417) (62.1515, -12.6194) (62.2396, -12.5974) (62.3279, -12.5758) (62.4163, -12.5545) (62.5049, -12.5334) (62.5936, -12.5127) (62.6824, -12.4923) (62.7714, -12.4721) (62.8605, -12.4523) (62.9497, -12.4328) (63.0391, -12.4135) (63.1286, -12.3946) (63.2182, -12.3759) (63.308, -12.3575) (63.3979, -12.3394) (63.4879, -12.3216) (63.578, -12.3041) (63.6683, -12.2869) (63.7586, -12.2699) (63.8491, -12.2532) (63.9216, -12.2401) (63.9761, -12.2304) (64.0124, -12.224) (64.0305, -12.2208) knots 0.405839 0.405839 0.405839 0.405839 0.405839 0.405839 0.414286 0.428571 0.442857 0.457143 0.471429 0.485714 0.5 0.514286 0.528571 0.542857 0.557143 0.571429 0.585714 0.6 0.614286 0.628571 0.642857 0.657143 0.671429 0.685714 0.7 0.714286 0.728571 0.742857 0.757143 0.771429 0.785714 0.8 0.814286 0.828571 0.842857 0.857143 0.871429 0.885714 0.9 0.914286 0.928571 0.942857 0.957143 0.971429 0.985714 1 1 1 1 1 1
  arc A73 (64.7457, -13.3335) -> (64.0305, -12.2208) centre (2.0032, -52.8695) ccw
  spline S74 degree 5 poles (64.7457, -13.3335) (64.7352, -13.3487) (64.7143, -13.3791) (64.6828, -13.4246) (64.6408, -13.485) (64.588, -13.5604) (64.535, -13.6356) (64.4819, -13.7105) (64.4285, -13.7852) (64.3749, -13.8597) (64.3211, -13.934) (64.2671, -14.008) (64.2129, -14.0818) (64.1585, -14.1553) (64.1038, -14.2286) (64.049, -14.3017) (63.9939, -14.3745) (63.9386, -14.4471) (63.8832, -14.5194) (63.8275, -14.5914) (63.7715, -14.6633) (63.7154, -14.7348) (63.6591, -14.8061) (63.6025, -14.8772) (63.5457, -14.9479) (63.4887, -15.0185) (63.4314, -15.0887) (63.374, -15.1587) (63.3163, -15.2284) (63.2583, -15.2978) (63.2002, -15.3669) (63.1418, -15.4358) (63.0832, -15.5043) (63.0243, -15.5726) (62.9652, -15.6406) (62.9059, -15.7082) (62.8463, -15.7756) (62.7865, -15.8427) (62.7264, -15.9094) (62.6661, -15.9758) (62.6055, -16.0419) (62.5447, -16.1077) (62.4886, -16.1678) (62.4446, -16.2146) (62.4127, -16.2482) (62.3931, -16.2688) (62.3858, -16.2765) knots -1 -1 -1 -1 -1 -1 -0.985714 -0.971429 -0.957143 -0.942857 -0.928571 -0.914286 -0.9 -0.885714 -0.871429 -0.857143 -0.842857 -0.828571 -0.814286 -0.8 -0.785714 -0.771429 -0.757143 -0.742857 -0.728571 -0.714286 -0.7 -0.685714 -0.671429 -0.657143 -0.642857 -0.628571 -0.614286 -0.6 -0.585714 -0.571429 -0.557143 -0.542857 -0.528571 -0.514286 -0.5 -0.485714 -0.471429 -0.457143 -0.442857 -0.428571 -0.414286 -0.405839 -0.405839 -0.405839 -0.405839 -0.405839 -0.405839
  arc A74 (63.0584, -17.4101) -> (62.3858, -16.2765) centre (2.0032, -52.8695) ccw
  spline S75 degree 5 poles (63.0584, -17.4101) (63.0686, -17.4074) (63.0961, -17.4) (63.1409, -17.3882) (63.2031, -17.372) (63.2827, -17.3516) (63.3696, -17.3297) (63.4566, -17.3082) (63.5438, -17.2871) (63.6312, -17.2664) (63.7187, -17.246) (63.8064, -17.226) (63.8942, -17.2063) (63.9822, -17.1871) (64.0703, -17.1681) (64.1586, -17.1495) (64.247, -17.1313) (64.3356, -17.1134) (64.4242, -17.0958) (64.5131, -17.0785) (64.602, -17.0616) (64.6911, -17.0451) (64.7803, -17.0288) (64.8697, -17.0129) (64.9591, -16.9973) (65.0487, -16.982) (65.1384, -16.967) (65.2282, -16.9523) (65.3182, -16.938) (65.4083, -16.924) (65.4984, -16.9102) (65.5887, -16.8968) (65.6791, -16.8837) (65.7697, -16.8709) (65.8603, -16.8583) (65.951, -16.8461) (66.0419, -16.8342) (66.1328, -16.8226) (66.2239, -16.8112) (66.315, -16.8002) (66.4063, -16.7894) (66.4976, -16.7789) (66.5891, -16.7687) (66.6623, -16.7608) (66.7173, -16.755) (66.754, -16.7512) (66.7723, -16.7493) knots 0.405839 0.405839 0.405839 0.405839 0.405839 0.405839 0.414286 0.428571 0.442857 0.457143 0.471429 0.485714 0.5 0.514286 0.528571 0.542857 0.557143 0.571429 0.585714 0.6 0.614286 0.628571 0.642857 0.657143 0.671429 0.685714 0.7 0.714286 0.728571 0.742857 0.757143 0.771429 0.785714 0.8 0.814286 0.828571 0.842857 0.857143 0.871429 0.885714 0.9 0.914286 0.928571 0.942857 0.957143 0.971429 0.985714 1 1 1 1 1 1
  arc A75 (67.4063, -17.9103) -> (66.7723, -16.7493) centre (2.0032, -52.8695) ccw
  spline S76 degree 5 poles (67.4063, -17.9103) (67.3948, -17.9247) (67.3717, -17.9535) (67.3371, -17.9966) (67.2908, -18.0539) (67.2328, -18.1253) (67.1746, -18.1965) (67.1162, -18.2675) (67.0577, -18.3382) (66.9989, -18.4087) (66.9399, -18.4789) (66.8808, -18.5489) (66.8215, -18.6186) (66.7619, -18.6881) (66.7022, -18.7573) (66.6423, -18.8262) (66.5822, -18.8949) (66.5219, -18.9634) (66.4614, -19.0316) (66.4007, -19.0995) (66.3398, -19.1671) (66.2787, -19.2345) (66.2174, -19.3016) (66.1559, -19.3684) (66.0942, -19.435) (66.0323, -19.5012) (65.9702, -19.5672) (65.9078, -19.6329) (65.8453, -19.6983) (65.7826, -19.7634) (65.7197, -19.8282) (65.6565, -19.8927) (65.5931, -19.9569) (65.5296, -20.0208) (65.4658, -20.0844) (65.4017, -20.1477) (65.3375, -20.2106) (65.2731, -20.2732) (65.2084, -20.3355) (65.1435, -20.3975) (65.0783, -20.4591) (65.013, -20.5203) (64.9528, -20.5763) (64.9055, -20.6198) (64.8713, -20.6511) (64.8503, -20.6703) (64.8425, -20.6774) knots -1 -1 -1 -1 -1 -1 -0.985714 -0.971429 -0.957143 -0.942857 -0.928571 -0.914286 -0.9 -0.885714 -0.871429 -0.857143 -0.842857 -0.828571 -0.814286 -0.8 -0.785714 -0.771429 -0.757143 -0.742857 -0.728571 -0.714286 -0.7 -0.685714 -0.671429 -0.657143 -0.642857 -0.628571 -0.614286 -0.6 -0.585714 -0.571429 -0.557143 -0.542857 -0.528571 -0.514286 -0.5 -0.485714 -0.471429 -0.457143 -0.442857 -0.428571 -0.414286 -0.405839 -0.405839 -0.405839 -0.405839 -0.405839 -0.405839
  arc A76 (65.4325, -21.8561) -> (64.8425, -20.6774) centre (2.0032, -52.8695) ccw
  spline S77 degree 5 poles (65.4325, -21.8561) (65.4429, -21.8541) (65.4708, -21.8487) (65.5163, -21.8401) (65.5795, -21.8284) (65.6604, -21.8137) (65.7486, -21.7981) (65.837, -21.7829) (65.9254, -21.768) (66.0141, -21.7536) (66.1028, -21.7395) (66.1917, -21.7258) (66.2807, -21.7125) (66.3698, -21.6995) (66.4591, -21.6869) (66.5485, -21.6746) (66.638, -21.6627) (66.7276, -21.6512) (66.8173, -21.64) (66.9071, -21.6291) (66.997, -21.6186) (67.0871, -21.6084) (67.1772, -21.5986) (67.2675, -21.5891) (67.3578, -21.5799) (67.4483, -21.571) (67.5388, -21.5625) (67.6295, -21.5543) (67.7202, -21.5464) (67.811, -21.5388) (67.902, -21.5315) (67.993, -21.5246) (68.0841, -21.518) (68.1753, -21.5116) (68.2666, -21.5056) (68.358, -21.4999) (68.4494, -21.4945) (68.541, -21.4894) (68.6326, -21.4845) (68.7243, -21.48) (68.8161, -21.4758) (68.908, -21.4719) (68.9999, -21.4682) (69.0736, -21.4656) (69.1288, -21.4637) (69.1657, -21.4625) (69.1841, -21.4619) knots 0.405839 0.405839 0.405839 0.405839 0.405839 0.405839 0.414286 0.428571 0.442857 0.457143 0.471429 0.485714 0.5 0.514286 0.528571 0.542857 0.557143 0.571429 0.585714 0.6 0.614286 0.628571 0.642857 0.657143 0.671429 0.685714 0.7 0.714286 0.728571 0.742857 0.757143 0.771429 0.785714 0.8 0.814286 0.828571 0.842857 0.857143 0.871429 0.885714 0.9 0.914286 0.928571 0.942857 0.957143 0.971429 0.985714 1 1 1 1 1 1
  arc A77 (69.7336, -22.6651) -> (69.1841, -21.4619) centre (2.0032, -52.8695) ccw
  spline S78 degree 5 poles (69.7336, -22.6651) (69.7211, -22.6787) (69.6961, -22.7058) (69.6585, -22.7463) (69.6082, -22.8002) (69.5453, -22.8673) (69.4821, -22.9341) (69.4188, -23.0008) (69.3553, -23.0671) (69.2917, -23.1332) (69.2279, -23.199) (69.1639, -23.2646) (69.0997, -23.3299) (69.0354, -23.395) (68.9709, -23.4598) (68.9062, -23.5243) (68.8414, -23.5885) (68.7763, -23.6525) (68.7111, -23.7162) (68.6457, -23.7796) (68.5801, -23.8427) (68.5144, -23.9055) (68.4485, -23.9681) (68.3824, -24.0304) (68.3161, -24.0923) (68.2496, -24.154) (68.1829, -24.2154) (68.1161, -24.2765) (68.0491, -24.3373) (67.9818, -24.3977) (67.9144, -24.4579) (67.8469, -24.5177) (67.7791, -24.5772) (67.7111, -24.6364) (67.6429, -24.6953) (67.5746, -24.7538) (67.506, -24.812) (67.4372, -24.8699) (67.3683, -24.9274) (67.2991, -24.9846) (67.2298, -25.0414) (67.1602, -25.0978) (67.0961, -25.1493) (67.0459, -25.1894) (67.0096, -25.2181) (66.9872, -25.2358) (66.9789, -25.2423) knots -1 -1 -1 -1 -1 -1 -0.985714 -0.971429 -0.957143 -0.942857 -0.928571 -0.914286 -0.9 -0.885714 -0.871429 -0.857143 -0.842857 -0.828571 -0.814286 -0.8 -0.785714 -0.771429 -0.757143 -0.742857 -0.728571 -0.714286 -0.7 -0.685714 -0.671429 -0.657143 -0.642857 -0.628571 -0.614286 -0.6 -0.585714 -0.571429 -0.557143 -0.542857 -0.528571 -0.514286 -0.5 -0.485714 -0.471429 -0.457143 -0.442857 -0.428571 -0.414286 -0.405839 -0.405839 -0.405839 -0.405839 -0.405839 -0.405839
  arc A78 (67.4833, -26.4601) -> (66.9789, -25.2423) centre (2.0032, -52.8695) ccw
  spline S79 degree 5 poles (67.4833, -26.4601) (67.4938, -26.4588) (67.5221, -26.4555) (67.5681, -26.4502) (67.632, -26.4429) (67.7137, -26.4341) (67.8028, -26.4248) (67.892, -26.4159) (67.9813, -26.4074) (68.0708, -26.3993) (68.1603, -26.3916) (68.2499, -26.3843) (68.3397, -26.3774) (68.4295, -26.3708) (68.5194, -26.3646) (68.6094, -26.3587) (68.6995, -26.3532) (68.7897, -26.3481) (68.88, -26.3433) (68.9704, -26.3389) (69.0608, -26.3348) (69.1514, -26.3311) (69.242, -26.3277) (69.3327, -26.3247) (69.4235, -26.322) (69.5143, -26.3196) (69.6052, -26.3175) (69.6962, -26.3158) (69.7873, -26.3144) (69.8785, -26.3133) (69.9697, -26.3126) (70.061, -26.3121) (70.1523, -26.312) (70.2438, -26.3122) (70.3352, -26.3127) (70.4268, -26.3135) (70.5184, -26.3146) (70.6101, -26.3161) (70.7018, -26.3178) (70.7936, -26.3198) (70.8855, -26.3222) (70.9774, -26.3248) (71.0694, -26.3277) (71.143, -26.3303) (71.1982, -26.3324) (71.2351, -26.3338) (71.2535, -26.3346) knots 0.405839 0.405839 0.405839 0.405839 0.405839 0.405839 0.414286 0.428571 0.442857 0.457143 0.471429 0.485714 0.5 0.514286 0.528571 0.542857 0.557143 0.571429 0.585714 0.6 0.614286 0.628571 0.642857 0.657143 0.671429 0.685714 0.7 0.714286 0.728571 0.742857 0.757143 0.771429 0.785714 0.8 0.814286 0.828571 0.842857 0.857143 0.871429 0.885714 0.9 0.914286 0.928571 0.942857 0.957143 0.971429 0.985714 1 1 1 1 1 1
  arc A79 (71.7158, -27.5739) -> (71.2535, -26.3346) centre (2.0032, -52.8695) ccw
  spline S80 degree 5 poles (71.7158, -27.5739) (71.7023, -27.5866) (71.6754, -27.6118) (71.635, -27.6495) (71.5811, -27.6997) (71.5135, -27.7621) (71.4458, -27.8243) (71.3779, -27.8862) (71.3098, -27.9479) (71.2416, -28.0093) (71.1733, -28.0704) (71.1048, -28.1312) (71.0361, -28.1918) (70.9673, -28.2521) (70.8983, -28.3121) (70.8292, -28.3718) (70.7599, -28.4313) (70.6905, -28.4905) (70.6209, -28.5493) (70.5512, -28.6079) (70.4813, -28.6662) (70.4112, -28.7242) (70.341, -28.7819) (70.2706, -28.8393) (70.2, -28.8964) (70.1293, -28.9531) (70.0585, -29.0096) (69.9874, -29.0658) (69.9163, -29.1216) (69.8449, -29.1771) (69.7734, -29.2323) (69.7017, -29.2872) (69.6298, -29.3417) (69.5578, -29.3959) (69.4856, -29.4498) (69.4132, -29.5033) (69.3407, -29.5564) (69.268, -29.6092) (69.1951, -29.6617) (69.1221, -29.7138) (69.0488, -29.7655) (68.9754, -29.8168) (68.9078, -29.8636) (68.8548, -29.9) (68.8166, -29.9261) (68.793, -29.9421) (68.7843, -29.948) knots -1 -1 -1 -1 -1 -1 -0.985714 -0.971429 -0.957143 -0.942857 -0.928571 -0.914286 -0.9 -0.885714 -0.871429 -0.857143 -0.842857 -0.828571 -0.814286 -0.8 -0.785714 -0.771429 -0.757143 -0.742857 -0.728571 -0.714286 -0.7 -0.685714 -0.671429 -0.657143 -0.642857 -0.628571 -0.614286 -0.6 -0.585714 -0.571429 -0.557143 -0.542857 -0.528571 -0.514286 -0.5 -0.485714 -0.471429 -0.457143 -0.442857 -0.428571 -0.414286 -0.405839 -0.405839 -0.405839 -0.405839 -0.405839 -0.405839
  arc A80 (69.2005, -31.1987) -> (68.7843, -29.948) centre (2.0032, -52.8695) ccw
  spline S81 degree 5 poles (69.2005, -31.1987) (69.2111, -31.1982) (69.2395, -31.1969) (69.2858, -31.1948) (69.35, -31.1922) (69.4321, -31.1891) (69.5217, -31.1862) (69.6113, -31.1838) (69.701, -31.1817) (69.7908, -31.18) (69.8806, -31.1787) (69.9706, -31.1778) (70.0606, -31.1772) (70.1506, -31.1771) (70.2408, -31.1773) (70.331, -31.1779) (70.4212, -31.1789) (70.5116, -31.1802) (70.602, -31.1819) (70.6924, -31.1839) (70.7829, -31.1863) (70.8735, -31.189) (70.9641, -31.1921) (71.0548, -31.1955) (71.1456, -31.1993) (71.2364, -31.2034) (71.3272, -31.2078) (71.4181, -31.2126) (71.509, -31.2177) (71.6, -31.2231) (71.6911, -31.2289) (71.7822, -31.235) (71.8733, -31.2414) (71.9645, -31.2481) (72.0557, -31.2551) (72.1469, -31.2624) (72.2382, -31.2701) (72.3296, -31.2781) (72.421, -31.2863) (72.5124, -31.2949) (72.6038, -31.3038) (72.6953, -31.313) (72.7869, -31.3225) (72.8601, -31.3303) (72.9151, -31.3363) (72.9517, -31.3404) (72.97, -31.3424) knots 0.405839 0.405839 0.405839 0.405839 0.405839 0.405839 0.414286 0.428571 0.442857 0.457143 0.471429 0.485714 0.5 0.514286 0.528571 0.542857 0.557143 0.571429 0.585714 0.6 0.614286 0.628571 0.642857 0.657143 0.671429 0.685714 0.7 0.714286 0.728571 0.742857 0.757143 0.771429 0.785714 0.8 0.814286 0.828571 0.842857 0.857143 0.871429 0.885714 0.9 0.914286 0.928571 0.942857 0.957143 0.971429 0.985714 1 1 1 1 1 1
  arc A81 (73.3427, -32.6116) -> (72.97, -31.3424) centre (2.0032, -52.8695) ccw